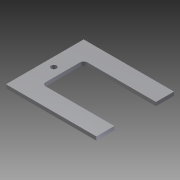
# Autodesk Inventor part: cetakan sepatu 2
Saved by Autodesk Inventor 2012 (Build 160160000, 160)
## iProperties
Created: 2014-01-20
Part Number: cetakan sepatu 2
Material: Default
Document SubType Name: Modeling
Designer: Irwan Haryanto
Density: 1 g/cm^3
Author: Irwan Haryanto
Autodesk Inventor part; units mm, degrees
ref_plane "YZ Plane" through (0, 0, 0) normal (1, 0, 0) x (0, 1, 0)
ref_plane "XZ Plane" through (0, 0, 0) normal (0, 1, 0) x (-1, 0, 0)
ref_plane "XY Plane" through (0, 0, 0) normal (0, 0, 1) x (1, 0, 0)
sketch "Sketch1" plane through (0, 0, 0) normal (0, 0, 1) x (1, 0, 0)
  circle A0 centre (-170.2692, -86.6522) radius 1.5
  line L0 (-175.2692, -65.1522) -> (-175.2692, -108.1522)
  arc A1 (-163.2692, -75.1522) -> (-165.2692, -77.1522) centre (-163.2692, -77.1522) ccw
  line L1 (-125.2692, -65.1522) -> (-175.2692, -65.1522)
  line L2 (-165.2692, -77.1522) -> (-165.2692, -96.1522)
  line L3 (-125.2692, -75.1522) -> (-125.2692, -65.1522)
  line L4 (-125.2692, -75.1522) -> (-163.2692, -75.1522)
  arc A2 (-165.2692, -96.1522) -> (-163.2692, -98.1522) centre (-163.2692, -96.1522) ccw
  line L5 (-175.2692, -108.1522) -> (-125.2692, -108.1522)
  line L6 (-125.2692, -108.1522) -> (-125.2692, -98.1522)
  line L7 (-163.2692, -98.1522) -> (-125.2692, -98.1522)
  point P0 (0, 0)
  point P1 (-165.2692, -75.1522)
  point P2 (-165.2692, -98.1522)
  dimension "d0" = 40
  dimension "d1" = 23
  dimension "d2" = 2
  dimension "d3" = 10
  dimension "d4" = 50
  dimension "d5" = 43
  dimension "d6" = 3
  dimension "d7" = 5
  dimension "d8" = 21.5
  constraints: 16 end point, 5 perpendicular, 4 point on circle, 4 point on line, 4 tangent, 3 centre point, 1 equal radius, 1 parallel
  measures "d0" distance of L3.start point (-165.269, -75.152)
  measures "d1" distance of point (-165.269, -75.152) point (-165.269, -98.152)
  measures "d2" radius of A1
  measures "d3" distance of L3.start L1.start
  measures "d4" distance of L1.start L1.end
  measures "d5" distance of L1.end L0.end
  measures "d6" diameter of A0
  measures "d7" distance from line of A0.centre L0
  measures "d8" distance from line of A0.centre L1
extrude "Extrusion1" add sketch "Sketch1" along normal blind 2
body "Solid1"
